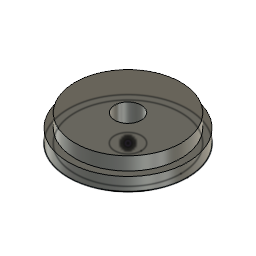
sprocket_9mm_2 (Autodesk Fusion 360 design; units mm, degrees)
Autodesk Fusion 360 part; units mm, degrees
sketch "スケッチ1" plane through (0, 0, 0) normal (0, 0, 1) x (1, 0, 0)
  circle A0 centre (0, 0) radius 4
  circle A1 centre (0, 0) radius 1
  circle A2 centre (0, 0) radius 4.5
  dimension "d1" = 8
  dimension "d2" = 2
  dimension "d5" = 9
  constraint coincident A0.centre A1.centre
  constraint concentric A0 A1
  constraint concentric A0 A2
  measures "d1" diameter of A0
  measures "d2" diameter of A1
  measures "d5" diameter of A2
extrude "押し出し1" add sketch "スケッチ1" along normal blind 2 contours A0 makes body 1
extrude "押し出し2" add sketch "スケッチ1" along normal blind 1 separate body contours A2 makes body 2
